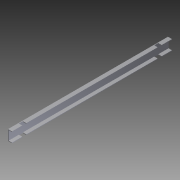
# Autodesk Inventor part: 2.25 U frame front
Saved by Autodesk Inventor 2012 (Build 160160000, 160)
## iProperties
Created: 2013-11-06
Part Number: 2.25 U frame front
Material: Default
Document SubType Name: Modeling
Designer: Bryce
Density: 1 g/cm^3
Author: Bryce
Autodesk Inventor part; units mm, degrees
ref_plane "YZ Plane" through (0, 0, 0) normal (1, 0, 0) x (0, 1, 0)
ref_plane "XZ Plane" through (0, 0, 0) normal (0, 1, 0) x (-1, 0, 0)
ref_plane "XY Plane" through (0, 0, 0) normal (0, 0, 1) x (1, 0, 0)
sketch "Sketch1" plane through (0, 0, 0) normal (0, 0, 1) x (1, 0, 0)
  line L0 (0, 0) -> (22.225, 0)
  line L1 (22.225, 0) -> (22.225, 57.15)
  line L2 (22.225, 57.15) -> (0, 57.15)
  line L3 (0, 57.15) -> (0, 0)
  line L4 (3.175, 3.175) -> (22.225, 3.175)
  line L5 (22.225, 3.175) -> (22.225, 53.975)
  line L6 (22.225, 53.975) -> (3.175, 53.975)
  line L7 (3.175, 53.975) -> (3.175, 3.175)
  dimension "d0" = 3.175
  dimension "d1" = 3.175
  dimension "d2" = 3.175
  dimension "d3" = 57.15
  dimension "d4" = 22.225
  constraints: 16 end point, 4 parallel, 2 horizontal, 2 perpendicular, 1 coincident, 1 point on line
  measures "d0" distance between parallel lines of L0 L4
  measures "d1" distance between parallel lines of L3 L7
  measures "d2" distance between parallel lines of L6 L2
  measures "d3" distance of L2.end L0.start
  measures "d4" distance of L0.start L0.end
extrude "Extrusion1" add sketch "Sketch1" along normal blind 889 contours L3 L2 L1 L6 L7 L4 L0
sketch "Sketch4" plane through (0, 57.15, 0) normal (0, 1, 0) x (1, 0, 0)
  line L0 (22.225, 0) -> (22.225, -889) projected
  line L1 (22.225, 0) -> (0, 0) projected
  line L2 (0, 0) -> (0, -889) projected
  line L3 (22.225, -57.15) -> (3.175, -57.15)
  line L4 (3.175, -57.15) -> (3.175, -79.375)
  line L5 (3.175, -79.375) -> (22.225, -79.375)
  line L6 (22.225, -79.375) -> (22.225, -57.15)
  line L7 (0, -444.5) -> (22.225, -444.5) construction
  line L8 (22.225, -831.85) -> (3.175, -831.85)
  line L9 (3.175, -831.85) -> (3.175, -809.625)
  line L10 (3.175, -809.625) -> (22.225, -809.625)
  line L11 (22.225, -809.625) -> (22.225, -831.85)
  dimension "d33" = 19.05
  dimension "d34" = 22.225
  dimension "d35" = 79.375
  dimension "d36" = 889
  dimension "d37" = 444.5
  constraints: 18 end point, 4 symmetric about line, 2 midpoint, 2 parallel, 2 perpendicular, 1 horizontal, 1 point on line
  measures "d33" distance of L3.start L3.end
  measures "d34" distance of L3.end L4.end
  measures "d35" distance between parallel lines of L1 L5
  measures "d36" distance of L1.end L2.end
  measures "d37" distance between parallel lines of L1 L7
extrude "Extrusion4" cut sketch "Sketch4" against normal through all
equation "\"d1\" = d0"
equation "\"d2\" = d0"
equation "\"d37\" = 0.5 * d36"
body "Solid1"
